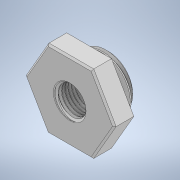
# Autodesk Inventor part: M24_2_1_4inch
Saved by Autodesk Inventor 2021 (Build 250183000, 183)
## iProperties
Created: 2021-01-28
Part Number: M24_2_1_4inch
Material: Generic
Document SubType Name: Modeling
Designer: Timo
Density: 1 g/cm^3
Appearance: Default
Author: Timo
Autodesk Inventor part; units mm, degrees
ref_plane "YZ Plane" through (0, 0, 0) normal (1, 0, 0) x (0, 1, 0)
ref_plane "XZ Plane" through (0, 0, 0) normal (0, 1, 0) x (-1, 0, 0)
ref_plane "XY Plane" through (0, 0, 0) normal (0, 0, 1) x (1, 0, 0)
sketch "Sketch1" plane through (0, 0, 0) normal (0, 0, 1) x (1, 0, 0)
  line L0 (-9.2376, 16) -> (9.2376, 16)
  line L1 (9.2376, 16) -> (18.4752, 0)
  line L2 (18.4752, 0) -> (9.2376, -16)
  line L3 (9.2376, -16) -> (-9.2376, -16)
  line L4 (-9.2376, -16) -> (-18.4752, 0)
  line L5 (-18.4752, 0) -> (-9.2376, 16)
  point P0 (0, 0)
  point P1 (0, 0)
  dimension "d0" = 32
  constraints: 12 end point, 1 coincident, 1 horizontal, 13 other
  measures "d0" distance between parallel lines of L3 L0
extrude "Extrusion1" add sketch "Sketch1" along normal blind 8
sketch "Sketch2" plane through (0, 0, 0) normal (0, 0, -1) x (-1, 0, 0)
  circle A0 centre (0, 0) radius 9.925
  dimension "d3" = 19.85
  constraints: 1 centre point, 1 coincident
  measures "d3" diameter of A0
extrude "Extrusion2" add sketch "Sketch2" along normal blind 8
sketch "Sketch3" plane through (0, 0, 0) normal (1, 0, 0) x (0, 1, 0)
  line L0 (9.925, 2.6258) -> (12.199, 1.3129)
  line L1 (12.199, 1.3129) -> (9.925, 0)
  line L2 (9.925, 0) -> (9.925, 2.6258)
  line L3 (11.75, 11.6995) -> (11.75, -11.0204) construction
  line L4 (10.9, -10.7686) -> (10.9, 10.1882) construction
  line L5 (9.925, 10.9583) -> (9.925, -10.6881) construction
  line L6 (16, 0) -> (0, 0) construction
  line L7 (11.75, 1.0537) -> (11.75, 1.5722)
  point P0 (10.9, 2.0629)
  point P1 (10.9, 0.5629)
  dimension "d6" = 19.85
  dimension "d7" = 21.8
  dimension "d8" = 23.5
  dimension "d9" = 30
  dimension "d10" = 60
  dimension "d11" = 1.5
  constraints: 14 end point, 11 point on line, 3 vertical
  measures "d6" diameter of L6.end L5
  measures "d7" diameter of L6.end L4
  measures "d8" diameter of L6.end L3
  measures "d9" angle of L6 L1
  measures "d10" angle of L1 L0
  measures "d11" distance of point (10.9, 2.063) point (10.9, 0.563)
coil "Coil1" sketch "Sketch3" operation add axis through (0, 0, -10) along (0, 0, -1) pitch 3 turns 5 hand right contours L0 L7 L1 L2
sketch "Sketch4" plane through (0, 0, -8) normal (0, 0, -1) x (-1, 0, 0)
  circle A0 centre (0, 0) radius 16.7379
  constraints: 1 centre point, 1 coincident
extrude "Extrusion3" cut sketch "Sketch4" along normal blind 8
sketch "Sketch5" plane through (0, 0, 0) normal (1, 0, 0) x (0, 1, 0)
  line L0 (11.8, -6.2) -> (10, -8)
  line L1 (10, -8) -> (11.8, -8)
  line L2 (11.8, -8) -> (11.8, -6.2)
  line L3 (11.6759, -8) -> (-4.9625, -8) projected
  line L4 (0, -9.6) -> (0, 1.6) projected
  point P0 (0, 0)
  dimension "d22" = 10
  dimension "d23" = 11.8
  dimension "d24" = 45
  constraints: 6 end point, 1 horizontal, 1 perpendicular, 1 point on line
  measures "d22" horizontal distance of point (0, 0) L0.end
  measures "d23" horizontal distance of point (0, 0) L1.end
  measures "d24" angle of L0 L1
revolve "Revolution1" cut sketch "Sketch5" angle 360 about axis through (0, 0, -10) along (0, 0, 1)
sketch "Sketch8" plane through (0, 0, 8) normal (0, 0, 1) x (1, 0, 0)
  circle A0 centre (0, 0) radius 5.7475
  dimension "d32" = 11.495
  constraints: 1 centre point, 1 coincident
  measures "d32" diameter of A0
extrude "Extrusion6" cut sketch "Sketch8" against normal through all
chamfer "Chamfer1" distance 1 angle 45 1 edges at (-5.7475, 0, 8)
sketch "Sketch10" plane through (0, 0, 0) normal (1, 0, 0) x (0, 1, 0)
  line L0 (5.7475, 19.2801) -> (5.7475, -12.7128) construction
  line L1 (6.175, 19.8987) -> (6.175, -12.7128) construction
  line L2 (6.6, 17.5481) -> (6.6, -10.4612) construction
  line L3 (6.7475, 8) -> (-6.7475, 8) projected
  line L4 (5.7475, 8) -> (6.817, 8.5568)
  line L5 (6.817, 8.5568) -> (5.7475, 9.1135)
  line L6 (5.7475, 8) -> (5.7475, 9.1135)
  line L7 (16, 8) -> (0, 8) projected
  line L8 (6.6, 8.6697) -> (6.6, 8.4438)
  point P0 (0, 0)
  point P1 (6.175, 8.891)
  point P2 (6.175, 8.2225)
  dimension "d38" = 5.7475
  dimension "d39" = 6.175
  dimension "d40" = 6.6
  dimension "d41" = 55
  dimension "d42" = 27.5
  dimension "d43" = 0.6684
  constraints: 14 end point, 11 point on line, 3 vertical, 1 perpendicular
  measures "d38" distance from line of point (0, 0) L0
  measures "d39" distance from line of point (0, 0) L1
  measures "d40" distance from line of point (0, 0) L2
  measures "d41" angle of L5 L4
  measures "d42" angle of L7 L4
  measures "d43" distance of point (6.175, 8.891) point (6.175, 8.223)
coil "Coil2" sketch "Sketch10" operation cut axis through (0, 0, -10) along (0, 0, -1) pitch 1.3368 turns 14.96063 hand right contours L6 L5 L8 L4
sketch "Sketch11" plane through (0, 0, -8) normal (0, 0, -1) x (-1, 0, 0)
  circle A0 centre (0, 0) radius 6.75
  dimension "d52" = 13.5
  constraints: 1 centre point, 1 coincident
  measures "d52" diameter of A0
extrude "Extrusion7" cut sketch "Sketch11" against normal blind 3
chamfer "Chamfer2" distance 0.7 angle 45 6 edges at (13.8564, 8, 8) (0, 16, 8) (-13.8564, 8, 8) (-13.8564, -8, 8) (0, -16, 8) (13.8564, -8, 8)
sketch "Sketch6" plane through (0, 0, 8) normal (0, 0, 1) x (1, 0, 0)
  circle A0 centre (0, 0) radius 9
  dimension "d26" = 18
  constraints: 1 centre point, 1 coincident
  measures "d26" diameter of A0
sketch "Sketch7" plane through (0, 0, 43) normal (0, 0, 1) x (1, 0, 0)
  circle A0 centre (0, 0) radius 9 projected
  circle A1 centre (0, 0) radius 7.5
  dimension "d29" = 1.5
  constraints: 1 centre point
  measures "d29" radial gap between concentric circles of A0 A1
equation "\"d42\" = 0.5 * d41"
body "Solid1"
